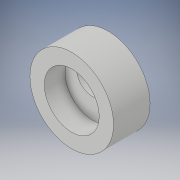
# Autodesk Inventor part: 30_raspi_lens_to_laser
Saved by Autodesk Inventor 2019 (Build 230136000, 136)
## iProperties
Created: 2020-09-01
Part Number: 30_raspi_lens_to_laser
Material: Generic
Document SubType Name: Modeling
Designer: marsikovabarbora
Density: 1 g/cm^3
Appearance: Default
Author: marsikovabarbora
Autodesk Inventor part; units mm, degrees
ref_plane "YZ Plane" through (0, 0, 0) normal (1, 0, 0) x (0, 1, 0)
ref_plane "XZ Plane" through (0, 0, 0) normal (0, 1, 0) x (-1, 0, 0)
ref_plane "XY Plane" through (0, 0, 0) normal (0, 0, 1) x (1, 0, 0)
sketch "Sketch1" plane through (0, 0, 0) normal (0, 0, 1) x (1, 0, 0)
  circle A0 centre (0, 0) radius 5.85 construction
  circle A1 centre (0, 0) radius 2.95 construction
  circle A2 centre (0, 0) radius 3.1
  circle A3 centre (0, 0) radius 8
  dimension "d0" = 11.7
  dimension "d1" = 5.9
  dimension "d2" = 6.2
  dimension "d3" = 16
  constraints: 4 centre point, 4 coincident
  measures "d0" diameter of A0
  measures "d1" diameter of A1
  measures "d2" diameter of A2
  measures "d3" diameter of A3
extrude "Extrusion1" add sketch "Sketch1" along normal blind 3 contours A2 | A3
sketch "Sketch2" plane through (0, 0, 3) normal (0, 0, 1) x (1, 0, 0)
  circle A0 centre (0, 0) radius 4.935 construction
  circle A1 centre (0, 0) radius 2.95 construction
  circle A2 centre (0, 0) radius 8 projected
  circle A3 centre (0, 0) radius 5.25
  dimension "d6" = 9.87
  dimension "d7" = 5.9
  dimension "d10" = 10.5
  constraints: 3 centre point, 3 coincident
  measures "d6" diameter of A0
  measures "d7" diameter of A1
  measures "d10" diameter of A3
extrude "Extrusion2" add sketch "Sketch2" along normal blind 4
sketch "Sketch3" plane through (0, 0, 0) normal (0, 0, -1) x (-1, 0, 0)
  circle A0 centre (0, 0) radius 8 construction
  circle A1 centre (0, 1.755) radius 3.1
  circle A2 centre (0, 0) radius 8 construction
  line L0 (0, -11.2) -> (0, 11.2) construction
  circle A3 centre (0, -2.095) radius 1.5 construction
  circle A4 centre (0, 1.755) radius 1.5 construction
  circle A5 centre (0, 0) radius 4.855 construction
  dimension "d13" = 6.2
  dimension "d14" = 3
  dimension "d15" = 3
  dimension "d16" = 3.85
  dimension "d21" = 9.71
  dimension "d22" = 1.6
  constraints: 4 centre point, 2 point on line, 1 coincident
  measures "d13" diameter of A1
  measures "d14" diameter of A3
  measures "d15" diameter of A4
  measures "d16" distance of A3.centre A1.centre
  measures "d21" diameter of A5
extrude "Extrusion3" cut sketch "Sketch3" against normal through all
body "Solid1"
